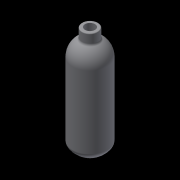
# Autodesk Inventor part: CO2Cartridge16g
Saved by Autodesk Inventor 2020.4 (Build 244396010, 396A)
## iProperties
Created: 2022-09-12
Part Number: CO2Cartridge16g
Material: Generic
Document SubType Name: Modeling
Designer: Val
Density: 1 g/cm^3
Appearance: Default
Author: Val
Autodesk Inventor part; units mm, degrees
ref_plane "YZ Plane" through (0, 0, 0) normal (1, 0, 0) x (0, 1, 0)
ref_plane "XZ Plane" through (0, 0, 0) normal (0, 1, 0) x (-1, 0, 0)
ref_plane "XY Plane" through (0, 0, 0) normal (0, 0, 1) x (1, 0, 0)
sketch "Sketch1" plane through (0, 0, 0) normal (0, 0, 1) x (1, 0, 0)
  line L0 (22.86, 101.6) -> (22.86, 12.7)
  line L1 (22.86, 101.6) -> (0, 101.6) construction
  line L2 (0, 101.6) -> (0, 12.7)
  line L3 (0, 12.7) -> (22.86, 12.7)
  line L4 (0, 101.6) -> (0, 122.1962)
  line L5 (0, 122.1962) -> (10.16, 122.1962) construction
  line L6 (10.16, 122.1962) -> (0, 122.1962)
  line L7 (0, 122.1962) -> (0, 134.8962)
  line L8 (0, 134.8962) -> (10.16, 134.8962)
  line L9 (10.16, 134.8962) -> (10.16, 122.1962)
  line L10 (0, 12.7) -> (0, 0)
  arc A0 (0, 0) -> (22.86, 12.7) centre (0, 26.924) ccw
  line L11 (0, 0) -> (22.86, 0) construction
  line L12 (22.86, 0) -> (22.86, 12.7) construction
  arc A1 (22.86, 101.6) -> (10.16, 122.1962) centre (-0.1909, 101.6) ccw
  point P0 (0, 122.1962)
  dimension "d0" = 88.9
  dimension "d1" = 22.86
  dimension "d3" = 10.16
  dimension "d4" = 12.7
  dimension "d5" = 12.7
  constraints: 26 end point, 4 horizontal, 4 point on circle, 4 vertical, 3 perpendicular, 2 centre point, 2 parallel, 2 tangent, 1 coincident, 1 collinear
  measures "d0" distance of L0.start L0.end
  measures "d1" distance of L0.start L1.end
  measures "d3" distance of L4.end L5.end
  measures "d4" distance of L8.end L5.end
  measures "d5" distance of L2.end L10.end
revolve "Revolution1" add sketch "Sketch1" angle 360 about axis through (0, 101.6, 0) along (0, -1, 0)
fillet "Fillet1" radius 6 1 edges at (-22.86, 12.7, 0)
fillet "Fillet2" radius 3.175 1 edges at (-10.16, 122.1962, 0)
sketch "Sketch2" plane through (0, 134.8962, 0) normal (0, 1, 0) x (1, 0, 0)
  circle A0 centre (0, 0) radius 10.16 projected
  circle A1 centre (0, 0) radius 6.35
  point P0 (0, 0)
  dimension "d9" = 12.7
  constraints: 1 centre point, 1 coincident
  measures "d9" diameter of A1
extrude "Extrusion1" cut sketch "Sketch2" against normal blind 25.4 contours A1
sketch "Sketch3" plane through (0, 109.4962, 0) normal (0, 1, 0) x (1, 0, 0)
  circle A0 centre (0, 0) radius 15.875
  dimension "d12" = 31.75
  constraints: 1 centre point, 1 coincident
  measures "d12" diameter of A0
extrude "Extrusion2" cut sketch "Sketch3" against normal blind 101.6
fillet "Fillet3" radius 6.35 2 edges at (-15.875, 109.4962, 0) (-15.875, 7.8962, 0)
fillet "Fillet4" radius 1 1 edges at (-10.16, 134.8962, 0)
body "Solid1"
